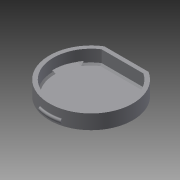
# Autodesk Inventor part: case_bottom
Saved by Autodesk Inventor 2015 (Build 190159000, 159)
## iProperties
Created: 2014-10-08
Part Number: case_bottom
Material: Generic
Document SubType Name: Modeling
Designer: Brad
Density: 1 g/cm^3
Appearance: Default
Author: Brad
Autodesk Inventor part; units mm, degrees
ref_plane "XZ Plane" through (0, 0, 0) normal (0, 1, 0) x (-1, 0, 0)
sketch "Sketch2" plane through (0, 0, 0) normal (0, 0, 1) x (1, 0, 0)
  line L0 (19.05, 5.11) -> (19.05, -6.0025)
  line L1 (19.05, -6.0025) -> (-19.05, -6.0025)
  line L2 (-19.05, -6.0025) -> (-19.05, 5.11)
  line L3 (11.43, -6.0025) -> (11.43, 1.9481)
  line L4 (-11.43, -6.0025) -> (-11.43, 1.5019)
  line L5 (16.51, 11.9875) -> (16.51, -11.3049)
  line L6 (-16.51, 11.9875) -> (-16.51, -11.3049)
  spline S0 degree 4 poles (11.43, -6.0025) (31.3158, 2.9384) (0, 13.9109) (-31.3158, 2.9384) (-11.43, -6.0025) knots 0 0 0 0 0 1 1 1 1 1
  line L7 (0, 5.9355) -> (0, -6.0025)
  line L8 (-16.51, 1.2137) -> (16.51, 1.2137)
  line L9 (0, 5.9355) -> (30.8491, 5.9355)
  point P0 (0, 0)
  dimension "d3" = 38.1
  dimension "d4" = 11.1125
  dimension "d5" = 38.1
  dimension "d6" = 19.05
  dimension "d8" = 11.43
  dimension "d9" = 16.51
  dimension "d54" = 16.51
  dimension "d113" = 11.938
  dimension "d114" = 5.9355
  constraints: 20 end point, 4 point on line, 2 horizontal, 2 perpendicular, 2 vertical, 1 midpoint, 1 parallel, 5 other
  measures "d3" distance of L2.end L0.start
  measures "d4" distance of L0.start L0.end
  measures "d5" distance of L0.end L1.end
  measures "d6" distance from line of point (0, 0) L0
  measures "d8" distance from line of L3 point (0, 0)
  measures "d9" distance from line of L5 point (0, 0)
  measures "d54" distance between parallel lines of L7 L6
  measures "d113" distance between parallel lines of L1 L9
  measures "d114" distance from line of point (0, 0) L9
revolve "Revolution1" add sketch "Sketch2" angle 360 about axis through (0, 5.9355, 0) along (0, -1, 0) picked at (5.3153, 2.7122) contours L1 L7 L8 L3 | L3 L8 L5 S0 | L8 L7 S0 | L5 S0
sketch "Sketch3" plane through (0, 0, 0) normal (1, 0, 0) x (0, 1, 0)
  point P0 (0, 0)
ref_plane "Work Plane1" through (0, 5.9355, 0) normal (0, -1, 0) x (1, 0, 0)
sketch "Sketch12" plane through (0, -6.0025, 0) normal (0, -1, 0) x (1, 0, 0)
  line L0 (0, 0) -> (0, -11.303)
  arc A0 (7.0756, -11.303) -> (-7.0756, -11.303) centre (0, 0) ccw
  line L1 (0, -11.303) -> (7.0756, -11.303)
  line L2 (0, -11.303) -> (-7.0756, -11.303)
  line L3 (22.0264, -21.1655) -> (-20.9628, -21.1655)
  line L4 (-20.9628, -21.1655) -> (-20.9628, 19.3861)
  line L5 (-20.9628, 19.3861) -> (22.0264, 19.3861)
  line L6 (22.0264, 19.3861) -> (22.0264, -21.1655)
  dimension "d42" = 11.303
  dimension "d43" = 26.67
  constraints: 14 end point, 3 horizontal, 2 parallel, 2 point on circle, 1 centre point, 1 coincident, 1 perpendicular, 1 vertical
  measures "d42" distance of L0.start L0.end
  measures "d43" diameter of A0
extrude "Extrusion9" cut sketch "Sketch12" against normal blind 25.4
sketch "Sketch15" plane through (1.6991, -6.0025, -11.303) normal (0, 0, -1) x (-1, 0, 0)
  line L0 (32.1125, 0) -> (-18.6875, 0)
  line L1 (-18.6875, 0) -> (-18.6875, 5.588)
  line L2 (-18.6875, 5.588) -> (32.1125, 5.588)
  line L3 (32.1125, 5.588) -> (32.1125, 0)
  line L4 (32.1125, 5.588) -> (32.1125, 12.4322)
  line L5 (32.1125, 12.4322) -> (-18.6875, 12.4322)
  line L6 (-18.6875, 12.4322) -> (-18.6875, 5.588)
  point P0 (1.6991, 6.0025)
  dimension "d69" = 5.588
  dimension "d75" = 50.8
  constraints: 14 end point, 5 perpendicular, 2 horizontal, 2 point on line
  measures "d69" distance of L0.end L1.end
  measures "d75" distance of L0.start L0.end
extrude "Extrusion10" cut sketch "Sketch15" against normal blind 50.8 contours L2 L6 L5 L4
sketch "Sketch16" plane through (-7.0756, -0.4145, -11.303) normal (0, 1, 0) x (1, 0, 0)
  arc A0 (0, 0) -> (14.1512, 0) centre (7.0756, -11.303) ccw
  line L0 (0, 0) -> (14.1512, 0)
  arc A1 (0.3746, -1.27) -> (13.7766, -1.27) centre (7.0756, -11.303) ccw
  line L1 (0.3746, -1.27) -> (13.7766, -1.27)
  point P0 (7.0756, -11.303)
  dimension "d72" = 1.27
  constraints: 4 end point, 4 point on circle, 2 centre point, 1 coincident, 1 horizontal, 1 other
  measures "d72" distance between parallel lines of L0 L1
extrude "Extrusion11" cut sketch "Sketch16" against normal blind 4.318 contours L1 A1
ref_plane "Work Plane8" through (0, -6.0025, 0) normal (0, 0, 1) x (1, 0, 0)
ref_plane "Work Plane7" through (0, -6.0025, -13.335) normal (0, 0, 1) x (1, 0, 0)
sketch "Sketch19" plane through (-1.6991, -6.0025, -11.303) normal (0, -1, 0) x (1, 0, 0)
  line L0 (1.6991, 11.303) -> (-11.6359, 11.303)
  line L1 (1.6991, 11.303) -> (-9.2242, 3.6544)
  line L2 (1.6991, 11.303) -> (-11.0187, 7.2931)
  circle A0 centre (1.6991, 11.303) radius 13.335
  line L3 (-11.0187, 7.2931) -> (-8.4411, -0.8821)
  arc A1 (8.7748, 0) -> (-5.3765, 0) centre (1.6991, 11.303) ccw projected
  line L4 (-11.0187, 7.2931) -> (-13.9992, 16.7461)
  line L5 (-11.6359, 11.303) -> (-12.2245, 11.1174)
  line L6 (-9.2242, 3.6544) -> (-9.8129, 3.4688)
  dimension "d104" = 35
  dimension "d105" = 17.5
  dimension "d106" = 26.67
  constraints: 14 end point, 3 point on circle, 2 perpendicular, 2 point on line, 2 tangent, 1 centre point, 1 coincident, 1 horizontal
  measures "d104" angle of L1 L0
  measures "d105" angle of L0 L2
  measures "d106" diameter of A0
ref_plane "Work Plane9" through (-12.7178, -6.0025, -4.0099) normal (-0.953717, 0, -0.3007058) x (0, -1, 0)
sketch "Sketch20" plane through (-12.7178, -6.0025, -4.0099) normal (-0.953717, 0, -0.3007058) x (0, -1, 0)
  line L0 (0, -10.2689) -> (0, 11.43) projected
  line L1 (0, 4.0392) -> (-1.27, 4.0392)
  line L2 (-1.27, -11.5837) -> (-1.27, 12.065) projected
  line L3 (0, -11.43) -> (0, -3.4371) projected
  line L4 (0, -4.016) -> (-1.27, -4.016)
  line L5 (-1.27, 4.0392) -> (-2.286, 4.0392)
  line L6 (-1.27, -4.016) -> (-2.286, -4.016)
  line L7 (-2.286, -4.016) -> (-2.286, 4.0392)
  line L8 (-1.27, 4.0392) -> (-1.27, -4.016)
  point P0 (-6.0025, 0)
  point P1 (-1.27, -7.5536)
  point P2 (0, -11.2908)
  dimension "d107" = 8.0552
  dimension "d108" = 1.016
  dimension "d109" = 1.016
  dimension "d115" = 1.27
  constraints: 12 end point, 4 point on line, 3 horizontal, 1 collinear, 1 parallel
  measures "d107" distance between parallel lines of L4 L1
  measures "d108" distance of L1.end L5.end
  measures "d109" distance of L4.end L6.end
  measures "d115" distance between parallel lines of L0 L2
extrude "Extrusion16" cut sketch "Sketch20" against normal blind 3.81 contours L6 L7 L5 L2
sketch "Sketch21" plane through (1.6991, -6.0025, -11.303) normal (0, 0, -1) x (-1, 0, 0)
  line L0 (8.7748, 5.588) -> (-5.3765, 5.588) projected
  line L1 (3.3983, 0) -> (0, 0) projected
  point P0 (1.6991, 6.0025)
  dimension "d112" = 5.588
  measures "d112" distance between parallel lines of L0 L1
sketch "Sketch22" plane through (0, 0, 0) normal (1, 0, 0) x (0, 1, 0)
  arc A0 (-4.4079, -11.303) -> (-4.4079, -11.303) centre (-3.7729, -11.303) ccw
  line L0 (-4.4079, -11.303) -> (-4.4079, -11.303)
  line L1 (-5.0429, -11.303) -> (-0.4145, -11.303) projected
  line L2 (-5.0429, -11.303) -> (-3.7729, -11.303)
  line L3 (-3.7729, -11.303) -> (-3.1379, -11.303)
  arc A1 (-4.4079, -11.303) -> (-3.1379, -11.303) centre (-3.7729, -11.303) ccw
  line L4 (-4.4079, -11.303) -> (-3.1379, -11.303)
  line L5 (-3.7729, -11.303) -> (-3.7729, -11.938)
  line L6 (-3.7729, -11.7602) -> (-4.768, -11.7602)
  arc A2 (-4.4079, -11.303) -> (-3.1379, -11.303) centre (-3.7729, -11.0906) ccw
  point P0 (0, 0)
  point P1 (-6.0025, -11.303)
  dimension "d122" = 1.27
  dimension "d124" = 1.27
  dimension "d130" = 0.4572
  constraints: 12 end point, 8 point on circle, 3 centre point, 3 point on line, 2 horizontal, 1 coincident, 1 collinear
  measures "d122" distance of L1.start L2.end
  measures "d124" diameter of A1
  measures "d130" distance between parallel lines of L1 L6
ref_plane "Work Plane10" through (0, -5.0429, 13.335) normal (0, 0, 1) x (1, 0, 0)
sketch "Sketch23" plane through (0, 0, 0) normal (1, 0, 0) x (0, 1, 0)
  line L0 (-5.0429, 13.335) -> (-0.4145, 13.335) projected
  line L1 (-5.0429, 13.335) -> (-3.7729, 13.335)
  line L2 (-4.4079, 13.335) -> (-3.1379, 13.335)
  line L3 (1.2005, 0) -> (-7.2032, 0) projected
  line L4 (-3.7729, 13.335) -> (-3.7729, 13.97)
  line L5 (-3.7729, 13.7922) -> (-3.0496, 13.7922)
  arc A0 (-3.1379, 13.335) -> (-4.4079, 13.335) centre (-3.7729, 13.1226) ccw
  line L6 (-4.4079, 13.335) -> (-3.1379, 13.335)
  line L7 (-4.4079, 13.335) -> (-3.1379, 13.335)
  line L8 (-5.0429, 13.335) -> (-0.4145, 13.335) projected
  point P0 (0, 0)
  dimension "d127" = 1.27
  dimension "d133" = 0.4572
  dimension "d134" = 0.6696
  dimension "d135" = 1.27
  constraints: 12 end point, 4 point on line, 3 point on circle, 2 horizontal, 1 centre point, 1 coincident, 1 collinear, 1 midpoint
  measures "d127" distance of L1.start L1.end
  measures "d133" distance between parallel lines of L0 L5
  measures "d134" radius of A0
  measures "d135" distance of L2.end L2.start
extrude "Extrusion19" add sketch "Sketch22" along normal mid plane 7.62 contours A2 L5 L1 | L1 L5 A2
revolve "Revolution8" add sketch "Sketch23" angle 30 mid plane about axis through (0, -6.0025, 0) along (0, -1, 0)
fillet "Fillet3" radius 0.254 6 edges at (0, -4.4079, 13.335) (0, -3.1379, 13.335) (1.905, -4.4079, -11.303) (-1.905, -4.4079, -11.303) (1.905, -3.1379, -11.303) (-1.905, -3.1379, -11.303)
chamfer "Chamfer1" distance 0.508 angle 45 3 edges at (5.8788, -4.7325, 10.5359) (0, -4.7325, -10.033) (-8.2894, -4.7325, -8.7664)
chamfer "Chamfer2" distance 0.762 angle 45 4 edges at (-10.2813, -4.7325, -7.4525) (-9.3852, -4.7325, -7.17) (-11.7994, -4.7325, 0.5149) (-12.6961, -4.7325, 0.2322)
body "Solid2"
